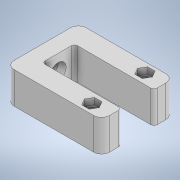
# Autodesk Inventor part: Tensor
Saved by Autodesk Inventor 2022 (Build 260153000, 153)
## iProperties
Created: 2022-03-05
Part Number: Tensor
Material: Genérico
Document SubType Name: Modeling
Designer: JK
Density: 1 g/cm^3
Appearance: Valor por defecto
Author: JK
Autodesk Inventor part; units mm, degrees
ref_plane "YZ Plane" through (0, 0, 0) normal (1, 0, 0) x (0, 1, 0)
ref_plane "XZ Plane" through (0, 0, 0) normal (0, 1, 0) x (-1, 0, 0)
ref_plane "XY Plane" through (0, 0, 0) normal (0, 0, 1) x (1, 0, 0)
sketch "Boceto1" plane through (0, 0, 0) normal (0, 1, 0) x (-1, 0, 0)
  line L0 (-5, 22.7) -> (5, 22.7)
  line L1 (5, 22.7) -> (5, -22.7)
  line L2 (5, -22.7) -> (-5, -22.7)
  line L3 (-5, -22.7) -> (-5, 22.7)
  line L4 (-5, 22.7) -> (5, -22.7) construction
  line L5 (5, 22.7) -> (-5, -22.7) construction
  line L6 (5, 22.7) -> (-55, 22.7)
  line L7 (-55, 22.7) -> (-55, 10.2)
  line L8 (-55, 10.2) -> (5, 10.2)
  line L9 (5, 10.2) -> (5, 22.7)
  line L10 (5, -22.7) -> (-55, -22.7)
  line L11 (-55, -22.7) -> (-55, -10.2)
  line L12 (-55, -10.2) -> (5, -10.2)
  line L13 (5, -10.2) -> (5, -22.7)
  point P0 (0, 0)
  point P1 (-5, 10.2)
  point P2 (-5, -10.2)
  point P3 (-5, -22.7)
  dimension "d0" = 20.4
  dimension "d1" = 45.4
  dimension "d2" = 60
  dimension "d3" = 10
  constraints: 28 end point, 6 parallel, 3 horizontal, 3 perpendicular, 2 midpoint, 1 collinear, 1 point on line
  measures "d0" distance between parallel lines of L12 L8
  measures "d1" distance of L0.end L1.end
  measures "d2" distance between parallel lines of L1 L7
  measures "d3" distance between parallel lines of L1 L3
extrude "Extrusión1" add sketch "Boceto1" along normal blind 20
sketch "Boceto2" plane through (-5, 0, -22.7) normal (-1, 0, 0) x (0, 0, 1)
  circle A0 centre (22.7, 10) radius 2.7
  line L0 (0, 0) -> (45.4, 0) projected
  point P0 (22.7, 0)
  dimension "d6" = 5.4
  dimension "d7" = 10
  constraints: 1 centre point
  measures "d6" diameter of A0
  measures "d7" distance from line of L0 A0.centre
extrude "Extrusión2" cut sketch "Boceto2" against normal through all
sketch "Boceto3" plane through (5, 0, 10.2) normal (1, 0, 0) x (0, 0, -1)
  point P0 (10.2, 0)
fillet "Empalme1" radius 5 2 edges at (-5, 10, -22.7) (-5, 10, 22.7)
sketch "Boceto4" plane through (0, 0, 0) normal (0, -1, 0) x (1, 0, 0)
  circle A0 centre (42.85, -16.7) radius 2.7
  circle A1 centre (42.85, 16.7) radius 2.7
  line L0 (55, -22.7) -> (0, -22.7) projected
  line L1 (0, 22.7) -> (55, 22.7) projected
  line L2 (55, 22.7) -> (55, 10.2) projected
  point P0 (0, 0)
  dimension "d11" = 6
  dimension "d12" = 6
  dimension "d13" = 5.4
  dimension "d19" = 12.15
  constraints: 2 centre point, 1 equal radius, 1 vertical alignment
  measures "d11" distance from line of L0 A0.centre
  measures "d12" distance from line of L1 A1.centre
  measures "d13" diameter of A0
  measures "d19" distance from line of L2 A1.centre
extrude "Extrusión3" cut sketch "Boceto4" against normal through all
sketch "Boceto5" plane through (0, 20, 0) normal (0, 1, 0) x (1, 0, 0)
  circle A0 centre (42.85, 16.7) radius 2.7 projected
  circle A1 centre (42.85, 16.7) radius 4.05
  circle A2 centre (42.85, -16.7) radius 2.7 projected
  circle A3 centre (42.85, -16.7) radius 4.05
  line L0 (47.5265, 16.7) -> (45.1883, 12.65)
  line L1 (45.1883, 12.65) -> (40.5117, 12.65)
  line L2 (40.5117, 12.65) -> (38.1735, 16.7)
  line L3 (38.1735, 16.7) -> (40.5117, 20.75)
  line L4 (40.5117, 20.75) -> (45.1883, 20.75)
  line L5 (45.1883, 20.75) -> (47.5265, 16.7)
  line L6 (47.5265, -7.8876) -> (52.82, -16.3438)
  line L7 (52.82, -16.3438) -> (48.1435, -25.1562)
  line L8 (48.1435, -25.1562) -> (38.1735, -25.5124)
  line L9 (38.1735, -25.5124) -> (32.88, -17.0562)
  line L10 (32.88, -17.0562) -> (37.5565, -8.2438)
  line L11 (37.5565, -8.2438) -> (47.5265, -7.8876)
  line L12 (40.5117, -20.75) -> (38.1735, -16.7)
  line L13 (38.1735, -16.7) -> (40.5117, -12.65)
  line L14 (40.5117, -12.65) -> (45.1883, -12.65)
  line L15 (45.1883, -12.65) -> (47.5265, -16.7)
  line L16 (47.5265, -16.7) -> (45.1883, -20.75)
  line L17 (45.1883, -20.75) -> (40.5117, -20.75)
  line L18 (0, -22.7) -> (55, -22.7) projected
  point P0 (0, 0)
  dimension "d16" = 8.1
  constraints: 36 end point, 5 coincident, 2 centre point, 2 tangent, 2 vertical alignment, 1 equal radius, 1 horizontal, 1 parallel, 39 other
  measures "d16" diameter of A1
extrude "Extrusión4" cut sketch "Boceto5" against normal blind 4 contours A0 | A1 | A1 L5 L0 | A1 L4 L5 | L0 L1 A1 | A1 L3 L4 | L1 L2 A1 | A1 L2 L3 | A2 | A3 | A3 L15 L16 | A3 L14 L15 | L16 L17 A3 | A3 L13 L14 | L17 L12 A3 | A3 L12 L13
fillet "Empalme2" radius 5 2 edges at (55, 10, 22.7) (55, 10, -22.7)
sketch "Boceto6" plane through (5, 0, 10.2) normal (1, 0, 0) x (0, 0, -1)
  circle A0 centre (10.2, 10) radius 2.7 projected
  circle A1 centre (10.2, 10) radius 5
  point P0 (10.2, 0)
  dimension "d21" = 10
  constraints: 1 centre point, 1 coincident
  measures "d21" diameter of A1
extrude "Extrusión5" cut sketch "Boceto6" against normal blind 5 contours A0 | A1
fillet "Empalme3" radius 2 4 edges at (5, 10, -10.2) (5, 10, 10.2) (55, 10, 10.2) (55, 10, -10.2)
